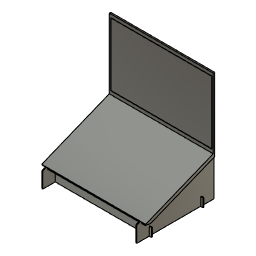
Laptop Stand (Autodesk Fusion 360 design; units mm, degrees)
Autodesk Fusion 360 part; units mm, degrees
note: some values were not read from the file. Set by a fixed rule: which sketch regions a step uses.
sketch "Sketch1" plane through (0, 0, 0) normal (1, 0, 0) x (0, 1, 0) in component "Leg"
  line L0 (0, 0) -> (269.9587, 0)
  line L1 (269.9587, 0) -> (269.9587, 147.8924)
  line L2 (269.9587, 147.8924) -> (19.6191, 46.7486)
  line L3 (19.6191, 46.7486) -> (14, 60.6564)
  line L4 (14, 60.6564) -> (0, 55)
  line L5 (0, 55) -> (0, 0)
  dimension "d1" = 22
  dimension "d3" = 14
  dimension "d4" = 55
  dimension "d40" = 270
  dimension "d41" = 15
  constraint coincident L0.start L5.end
  constraint horizontal L0
  constraint perpendicular L0 L1
  constraint perpendicular L2 L3
  constraint perpendicular L3 L4
  constraint vertical L5
  measures "d1" angle of L0 L2
  measures "d3" horizontal distance of L3.end L4.end
  measures "d4" distance of L4.end L0.start
  measures "d40" distance of L1.end L2.end
  measures "d41" distance of L2.end L3.end
extrude "Extrude1" add sketch "Sketch1" along normal blind 3 makes body 1 in component "Leg"
fillet "Fillet1" radius 3 4 edges at (1.5, 0, 55) (1.5, 14, 60.6564) (1.5, 19.6191, 46.7486) (1.5, 269.9587, 147.8924) on bodies 1 in component "Leg"
sketch "Sketch1 (2)" plane through (0, -13.484, 33.3741) normal (0, -0.374607, 0.927184) x (1, 0, 0) in component "Top"
  line L0 (3, 301.2552) -> (0, 301.2552)
  line L1 (0, 301.2552) -> (0, 38.7028)
  line L2 (0, 38.7028) -> (3, 38.7028)
  line L3 (3, 38.7028) -> (3, 301.2552)
  line L4 (-325, 301.2552) -> (-328, 301.2552)
  line L5 (-328, 301.2552) -> (-328, 38.7028)
  line L6 (-328, 38.7028) -> (-325, 38.7028)
  line L7 (-325, 38.7028) -> (-325, 301.2552)
  line L8 (-336, 289.2552) -> (11, 289.2552)
  line L9 (11, 289.2552) -> (11, 38.7028)
  line L10 (11, 38.7028) -> (-336, 38.7028)
  line L11 (-336, 38.7028) -> (-336, 289.2552)
  line L12 (0, 259.2552) -> (3, 259.2552)
  line L13 (3, 259.2552) -> (3, 234.2552)
  line L14 (3, 234.2552) -> (0, 234.2552)
  line L15 (0, 234.2552) -> (0, 259.2552)
  line L16 (-162.5, 289.2552) -> (-162.5, 38.7028) construction
  line L17 (-336, 163.979) -> (11, 163.979) construction
  line L18 (-328, 259.2552) -> (-328, 234.2552)
  line L19 (-325, 234.2552) -> (-325, 259.2552)
  line L20 (-325, 259.2552) -> (-328, 259.2552)
  line L21 (-328, 234.2552) -> (-325, 234.2552)
  line L22 (3, 68.7028) -> (3, 93.7028)
  line L23 (0, 93.7028) -> (0, 68.7028)
  line L24 (3, 93.7028) -> (0, 93.7028)
  line L25 (0, 68.7028) -> (3, 68.7028)
  line L26 (-325, 68.7028) -> (-328, 68.7028)
  line L27 (-328, 68.7028) -> (-328, 93.7028)
  line L28 (-325, 93.7028) -> (-325, 68.7028)
  line L29 (-328, 93.7028) -> (-325, 93.7028)
  dimension "d23" = 12
  dimension "d24" = 8
  dimension "d25" = 8
  dimension "d26" = 25
  dimension "d27" = 30
  constraint horizontal L8
  constraint vertical L9
  constraint horizontal L10
  constraint vertical L11
  constraint collinear L2 L10
  constraint horizontal L12
  constraint vertical L13
  constraint horizontal L14
  constraint vertical L15
  constraint coincident L3 L13.end
  constraint coincident L1 L12.start
  constraint midpoint L8 L16.start
  constraint midpoint L10 L16.end
  constraint midpoint L11 L17.start
  constraint midpoint L9 L17.end
  constraint symmetric L12.start L16 L19.end
  constraint symmetric L12.end L16 L18.start
  constraint symmetric L13.end L16 L18.end
  constraint symmetric L14.end L16 L19.start
  constraint symmetric L12.start L17 L23.end
  constraint symmetric L12.end L17 L22.start
  constraint symmetric L13.end L17 L22.end
  constraint symmetric L14.end L17 L23.start
  constraint symmetric L17 L18.start L26.end
  constraint symmetric L17 L18.end L27.end
  constraint symmetric L17 L19.start L28.start
  constraint symmetric L17 L19.end L26.start
  measures "d23" distance of L0.start L8
  measures "d24" distance of L3 L8.end
  measures "d25" distance of L5 L11
  measures "d26" distance of L12 L14
  measures "d27" distance of L8 L12
extrude "Extrude1'" add sketch "Sketch1 (2)" against normal blind 3 separate body contours L3 L8 L9 L10 L13 L22 | L1 L3 L8 L12 | L1 L7 L8 L10 L15 L19 L23 L28 | L5 L7 L8 L20 | L1 L3 L14 L24 | L5 L8 L10 L11 L18 L27 | L1 L2 L3 L10 L25 | L5 L7 L21 L29 | L5 L6 L7 L10 L26 makes body 2 in component "Top"
combine "Combine1" operation cut target body 1 tool bodies 2 keep tools in component "Leg"
fillet "Fillet1'" radius 2 4 edges at (-336, 22.9626, 46.4817) (11, 22.9626, 46.4817) (11, 255.2706, 140.3402) (-336, 255.2706, 140.3402) on bodies 2 in component "Top"
ref_plane "WorkPlane1" through (1.5, 224.9587, 73.9462) normal (0, 1, 0) x (0, 0, 1) in component "Support"
sketch "Sketch1 (3)" plane through (1.5, 224.9587, 60.2762) normal (0, 1, 0) x (1, 0, 0) in component "Support"
  line L0 (-329.5, -69.4351) -> (-326.5, -69.4351)
  line L1 (-326.5, -69.4351) -> (-326.5, 60.2762)
  line L2 (-326.5, 60.2762) -> (-329.5, 60.2762)
  line L3 (-329.5, 60.2762) -> (-329.5, -69.4351)
  line L4 (-1.5, -69.4351) -> (1.5, -69.4351)
  line L5 (1.5, -69.4351) -> (1.5, 60.2762)
  line L6 (1.5, 60.2762) -> (-1.5, 60.2762)
  line L7 (-1.5, 60.2762) -> (-1.5, -69.4351)
  line L8 (9.5, 60.2762) -> (-337.5, 60.2762)
  line L9 (-337.5, 60.2762) -> (-337.5, 30.2762)
  line L10 (-337.5, 30.2762) -> (9.5, 30.2762)
  line L11 (9.5, 30.2762) -> (9.5, 60.2762)
  line L12 (-337.5, 14.4361) -> (-337.5, -77.9241)
  line L13 (9.5, -77.9241) -> (9.5, 14.4361)
  line L14 (9.5, 45.2762) -> (-337.5, 45.2762)
  dimension "d32" = 30
  constraint horizontal L8
  constraint vertical L9
  constraint horizontal L10
  constraint vertical L11
  constraint collinear L2 L8
  constraint collinear L9 L12
  constraint collinear L11 L13
  constraint midpoint L11 L14.start
  constraint midpoint L9 L14.end
  measures "d32" distance of L8.start L10.end
extrude "Extrude1''" add sketch "Sketch1 (3)" along normal mid plane 3 separate body contours L3 L9 L10 L14 | L1 L7 L10 L14 | L3 L8 L9 L14 | L1 L2 L3 L8 L14 | L1 L7 L8 L14 | L5 L6 L7 L8 L14 | L5 L10 L11 L14 | L5 L8 L11 L14 makes body 3 in component "Support"
ref_plane "WorkPlane2" through (1.5, 134.9794, 73.9462) normal (0, 1, 0) x (0, 0, 1) in component "Support"
mirror "Mirror1" about plane through (1.5, 134.9794, 73.9462) normal (0, 1, 0) of bodies 3 makes body 4 in component "Support"
fillet "Fillet1''" radius 2 2 edges at (11, 224.9587, 30) (-336, 224.9587, 30) on bodies 3 4 in component "Support"
fillet "Fillet1''" radius 2 2 edges at (11, 45, 30) (-336, 45, 30) on bodies 3 4 in component "Support"
fillet "Fillet2" radius 0.5 4 edges at (-328, 224.9587, 30) (-325, 224.9587, 30) (0, 224.9587, 30) (3, 224.9587, 30) on bodies 3 in component "Support"
combine "Combine2" operation cut target body 1 tool bodies 4 3 keep tools in component "Leg"
fillet "Fillet2'" radius 0.5 10 edges at (3, 134.9794, 0) (1.5, 226.4587, 0) (1.5, 43.5, 0) (1.5, 46.5, 0) (1.5, 22.4007, 47.8724) (1.5, 50.2162, 59.1106) (1.5, 73.3958, 68.4758) (1.5, 203.7136, 121.1276) (1.5, 226.8932, 130.4928) (1.5, 254.7087, 141.731) on bodies 1 in component "Leg"
sketch "Side DXF" plane through (3, 0, 0) normal (1, 0, 0) x (0, 1, 0)
  arc A0 (255.1723, 141.9183) -> (254.896, 141.2674) centre (255.3596, 141.4547) ccw
  line L0 (254.896, 141.2674) -> (255.8325, 138.9494)
  line L1 (255.8325, 138.9494) -> (228.017, 127.7112)
  line L2 (228.017, 127.7112) -> (227.0805, 130.0292)
  arc A1 (227.0805, 130.0292) -> (226.4296, 130.3055) centre (226.6169, 129.8419) ccw
  line L3 (226.4296, 130.3055) -> (204.1772, 121.3149)
  arc A2 (204.1772, 121.3149) -> (203.9009, 120.664) centre (204.3645, 120.8513) ccw
  line L4 (203.9009, 120.664) -> (204.8374, 118.3461)
  line L5 (204.8374, 118.3461) -> (74.5196, 65.6942)
  line L6 (74.5196, 65.6942) -> (73.5831, 68.0122)
  arc A3 (73.5831, 68.0122) -> (72.9322, 68.2885) centre (73.1195, 67.8249) ccw
  line L7 (72.9322, 68.2885) -> (50.6798, 59.2979)
  arc A4 (50.6798, 59.2979) -> (50.4035, 58.647) centre (50.8671, 58.8343) ccw
  line L8 (50.4035, 58.647) -> (51.34, 56.3291)
  line L9 (51.34, 56.3291) -> (23.5245, 45.0909)
  line L10 (23.5245, 45.0909) -> (22.5745, 47.4421)
  arc A5 (22.5745, 47.4421) -> (21.9918, 47.7404) centre (22.1109, 47.2548) ccw
  arc A6 (18.4953, 49.5302) -> (21.9918, 47.7404) centre (21.2768, 50.654) ccw
  line L11 (18.4953, 49.5302) -> (15.1238, 57.8748)
  arc A7 (15.1238, 57.8748) -> (11.2184, 59.5325) centre (12.3423, 56.751) ccw
  line L12 (11.2184, 59.5325) -> (1.8762, 55.758)
  arc A8 (1.8762, 55.758) -> (0, 52.9765) centre (3, 52.9765) ccw
  line L13 (0, 52.9765) -> (0, 0)
  line L14 (0, 0) -> (43, 0)
  arc A9 (43, 0) -> (43.5, 0.5) centre (43, 0.5) ccw
  line L15 (43.5, 0.5) -> (43.5, 15)
  line L16 (43.5, 15) -> (46.5, 15)
  line L17 (46.5, 15) -> (46.5, 0.5)
  line L18 (46.5, 0.5) -> (223.4587, 0.5)
  line L19 (223.4587, 0.5) -> (223.4587, 15)
  line L20 (223.4587, 15) -> (226.4587, 15)
  line L21 (226.4587, 15) -> (226.4587, 0.5)
  arc A10 (226.4587, 0.5) -> (226.9587, 0) centre (226.9587, 0.5) ccw
  line L22 (226.9587, 0) -> (269.9587, 0)
  line L23 (269.9587, 0) -> (269.9587, 143.4447)
  arc A11 (269.9587, 143.4447) -> (265.8349, 146.2263) centre (266.9587, 143.4447) ccw
  line L24 (265.8349, 146.2263) -> (255.1723, 141.9183)
sketch "Top DXF" plane through (0, -13.484, 33.3741) normal (0, -0.374607, 0.927184) x (1, 0, 0)
  line L0 (-325, 234.2552) -> (-328, 234.2552)
  line L1 (-328, 234.2552) -> (-328, 259.2552)
  line L2 (-328, 259.2552) -> (-325, 259.2552)
  line L3 (-325, 259.2552) -> (-325, 234.2552)
  line L4 (-328, 68.7028) -> (-328, 93.7028)
  line L5 (-328, 93.7028) -> (-325, 93.7028)
  line L6 (-325, 93.7028) -> (-325, 68.7028)
  line L7 (-325, 68.7028) -> (-328, 68.7028)
  line L8 (3, 234.2552) -> (0, 234.2552)
  line L9 (0, 234.2552) -> (0, 259.2552)
  line L10 (0, 259.2552) -> (3, 259.2552)
  line L11 (3, 259.2552) -> (3, 234.2552)
  line L12 (3, 68.7028) -> (0, 68.7028)
  line L13 (0, 68.7028) -> (0, 93.7028)
  line L14 (0, 93.7028) -> (3, 93.7028)
  line L15 (3, 93.7028) -> (3, 68.7028)
  arc A0 (-334, 289.2552) -> (-336, 287.2552) centre (-334, 287.2552) ccw
  line L16 (-336, 287.2552) -> (-336, 40.7028)
  arc A1 (-336, 40.7028) -> (-334, 38.7028) centre (-334, 40.7028) ccw
  line L17 (-334, 38.7028) -> (9, 38.7028)
  arc A2 (9, 38.7028) -> (11, 40.7028) centre (9, 40.7028) ccw
  line L18 (11, 40.7028) -> (11, 287.2552)
  arc A3 (11, 287.2552) -> (9, 289.2552) centre (9, 287.2552) ccw
  line L19 (9, 289.2552) -> (-334, 289.2552)
sketch "Support DXF" plane through (0, 43.5, 0) normal (0, -1, 0) x (1, 0, 0)
  line L0 (11, 0) -> (11, 28)
  line L1 (9, 30) -> (3, 30)
  line L2 (3, 30) -> (3, 15)
  line L3 (3, 15) -> (0, 15)
  line L4 (0, 15) -> (0, 30)
  line L5 (0, 30) -> (-325, 30)
  line L6 (-325, 30) -> (-325, 15)
  line L7 (-325, 15) -> (-328, 15)
  line L8 (-328, 15) -> (-328, 30)
  line L9 (-328, 30) -> (-334, 30)
  line L10 (-336, 28) -> (-336, 0)
  line L11 (-336, 0) -> (11, 0)
  arc A0 (-334, 30) -> (-336, 28) centre (-334, 28) ccw
  arc A1 (11, 28) -> (9, 30) centre (9, 28) ccw
sketch "Sketch1 (4)" plane through (0, -13.484, 33.3741) normal (0, -0.374607, 0.927184) x (1, 0, 0) in component "Laptop"
  line L0 (-344, 290.7028) -> (19, 290.7028)
  line L1 (19, 290.7028) -> (19, 35.7028)
  line L2 (19, 35.7028) -> (-344, 35.7028)
  line L3 (-344, 35.7028) -> (-344, 290.7028)
  line L4 (-334, 38.7028) -> (9, 38.7028)
  line L5 (9, 289.2552) -> (-334, 289.2552)
  line L6 (-162.5, 289.2552) -> (-162.5, 35.7028) construction
  point P0 (3, 35.7028)
  dimension "d42" = 255
  dimension "d43" = 363
  constraint horizontal L0
  constraint vertical L1
  constraint horizontal L2
  constraint vertical L3
  constraint coincident L2 P0
  constraint midpoint L5 L6.start
  constraint midpoint L2 L6.end
  constraint vertical L6
  measures "d42" distance of L0.start L2.end
  measures "d43" distance of L0.start L0.end
extrude "Extrude1'''" add sketch "Sketch1 (4)" along normal blind 12 separate body makes body 5 in component "Laptop"
chamfer "Chamfer1" distance 14 distance2 9 1 edges at (-162.5, 19.6191, 46.7486) measured on face at (-223, 98.4297, 78.5902) on bodies 5 in component "Laptop"
ref_plane "WorkPlane1" through (0, 0, 142.273) normal (0, 0, 1) x (1, 0, 0)
sketch "Sketch4" plane through (0, 0, 142.273) normal (0, 0, 1) x (1, 0, 0)
  line L0 (-344, 256.051) -> (19, 256.051)
  line L1 (19, 256.051) -> (-344, 256.051)
  line L2 (-344, 256.051) -> (-344, 251.051)
  line L3 (-344, 251.051) -> (19, 251.051)
  line L4 (19, 251.051) -> (19, 256.051)
  dimension "d49" = 5
  constraint horizontal L1
  constraint vertical L2
  constraint horizontal L3
  constraint vertical L4
  constraint coincident L0.end L1.start
  measures "d49" distance of L0.start L2.end
extrude "Extrude1''''" add sketch "Sketch4" along normal blind 255 separate body makes body 6
combine "Combine1'" operation add target body 6 tool bodies 5
sketch "Sketch5" plane through (0, 251.051, 0) normal (0, -1, 0) x (1, 0, 0)
  line L0 (-344, 153.1956) -> (19, 153.1956)
  line L1 (19, 153.1956) -> (19, 397.273)
  line L2 (19, 397.273) -> (-344, 397.273)
  line L3 (-344, 397.273) -> (-344, 153.1956)
  line L4 (-339, 385.273) -> (14, 385.273)
  line L5 (14, 385.273) -> (14, 165.1956)
  line L6 (14, 165.1956) -> (-339, 165.1956)
  line L7 (-339, 165.1956) -> (-339, 385.273)
  dimension "d52" = 5
  dimension "d53" = 5
  dimension "d54" = 12
  dimension "d55" = 12
  constraint horizontal L4
  constraint vertical L5
  constraint horizontal L6
  constraint vertical L7
  measures "d52" distance of L3 L7
  measures "d53" distance of L1 L5
  measures "d54" distance of L2 L4
  measures "d55" distance of L0 L6
extrude "Extrude2" cut sketch "Sketch5" against normal blind 1 contours L4 L5 L6 L7 bodies 6
copy_body "CutPasteBodies1" bodies 6 removing the originals makes body 7 in component "Laptop"
component "Leg" placed x (1, 0, 0) y (0, 1, 0) z (0, 0, 1) at (0, 0, 0)
component "Leg" placed x (1, 0, 0) y (0, 1, 0) z (0, 0, 1) at (-328, 0, 0)
component "Top" placed x (1, 0, 0) y (0, 1, 0) z (0, 0, 1) at (0, 0, 0)
component "Support" placed x (1, 0, 0) y (0, 1, 0) z (0, 0, 1) at (0, 0, 0)
component "Laptop" placed x (1, 0, 0) y (0, 1, 0) z (0, 0, 1) at (0, 0, 0)
equation "t = 3 mm" comment "Material Thickness"
equation "w = 325 mm" comment "Leg Width"
equation "d8 = t"
equation "d22 = w"
equation "d28 = -t"
equation "d33 = ( t / 2 mm ) * 1 mm"
equation "L = 270 mm" comment "Length"
equation "d40 = L"
